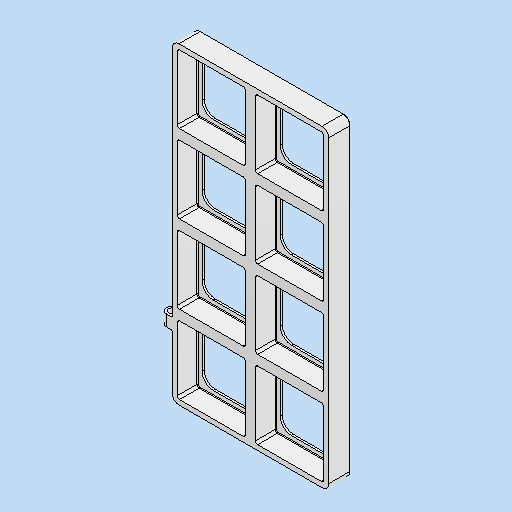
# Autodesk Inventor part: SampleCell
Saved by Autodesk Inventor 2025 (Build 290162000, 162)
## iProperties
Created: 2024-10-28
Part Number: SampleCell
Material: ABS Plastic
Document SubType Name: Modeling
Designer: kuzmin
Density: 1.06 g/cm^3
Appearance: Smooth - White
Author: kuzmin
Autodesk Inventor part; units mm, degrees
ref_plane "YZ Plane" through (0, 0, 0) normal (1, 0, 0) x (0, 1, 0)
ref_plane "XZ Plane" through (0, 0, 0) normal (0, 1, 0) x (-1, 0, 0)
sketch "Sketch1" plane through (0, 0, 0) normal (0, 0, 1) x (-1, 0, 0)
  line L0 (17.5, 17.5) -> (-17.5, 17.5)
  line L1 (-17.5, 17.5) -> (-17.5, -17.5)
  line L2 (-17.5, -17.5) -> (17.5, -17.5)
  line L3 (17.5, -17.5) -> (17.5, 17.5)
  point P0 (0, 0)
  point P1 (17.5, 0)
  point P2 (0, -17.5)
  dimension "d0" = 35
  constraints: 8 end point, 2 midpoint, 2 parallel, 2 perpendicular, 1 horizontal, 1 horizontal alignment, 1 vertical alignment
  measures "d0" distance of L2.end L0.start
extrude "Extrusion1" add sketch "Sketch1" along normal blind 10
sketch "Sketch2" plane through (0, 0, 10) normal (0, 0, 1) x (1, 0, 0)
  line L0 (-15.25, -15.25) -> (15.25, -15.25)
  line L1 (15.25, -15.25) -> (15.25, 15.25)
  line L2 (15.25, 15.25) -> (-15.25, 15.25)
  line L3 (-15.25, 15.25) -> (-15.25, -15.25)
  point P0 (0, 0)
  point P1 (-15.25, 0)
  point P2 (0, 15.25)
  dimension "d3" = 30.5
  constraints: 8 end point, 2 midpoint, 2 parallel, 2 perpendicular, 1 horizontal, 1 horizontal alignment, 1 vertical alignment
  measures "d3" distance of L2.end L0.start
extrude "Extrusion2" cut sketch "Sketch2" against normal through all
sketch "Sketch3" plane through (0, 0, 0) normal (0, 0, -1) x (1, 0, 0)
  line L0 (15.25, 15.25) -> (15.25, -15.25) projected
  line L1 (-15.25, 15.25) -> (15.25, 15.25) projected
  line L2 (-15.25, -15.25) -> (-15.25, 15.25) projected
  line L3 (15.25, -15.25) -> (-15.25, -15.25) projected
  line L4 (13.25, 13.25) -> (-13.25, 13.25)
  line L5 (-13.25, 13.25) -> (-13.25, -13.25)
  line L6 (-13.25, -13.25) -> (13.25, -13.25)
  line L7 (13.25, -13.25) -> (13.25, 13.25)
  point P0 (0, 0)
  point P1 (13.25, 0)
  point P2 (0, -13.25)
  dimension "d6" = 2
  constraints: 8 end point, 2 midpoint, 2 parallel, 2 perpendicular, 1 horizontal, 1 horizontal alignment, 1 vertical alignment
  measures "d6" distance between parallel lines of L0 L7
extrude "Extrusion3" add sketch "Sketch3" against normal blind 0.9
fillet "Fillet1" radius 1 4 edges at (-15.25, -15.25, 5.45) (-15.25, 15.25, 5.45) (15.25, 15.25, 5.45) (15.25, -15.25, 5.45)
fillet "Fillet2" radius 5 4 edges at (-13.25, -13.25, 0.45) (-13.25, 13.25, 0.45) (13.25, 13.25, 0.45) (13.25, -13.25, 0.45)
chamfer "Chamfer1" distance 0.3 angle 45 8 edges at (0, 15.25, 0.9) (14.9571, 14.9571, 0.9) (15.25, 0, 0.9) (14.9571, -14.9571, 0.9) (0, -15.25, 0.9) (-14.9571, -14.9571, 0.9) (-15.25, 0, 0.9) (-14.9571, 14.9571, 0.9)
pattern_linear "Rectangular Pattern1" count 2 spacing 35 along (1, 0, 0) count 4 spacing 35 along (0, 1, 0)
fillet "Fillet4" radius 3 4 edges at (52.5, 122.5, 5) (-17.5, 122.5, 5) (52.5, -17.5, 5) (-17.5, -17.5, 5)
chamfer "Chamfer2" distance 0.5 angle 45 8 edges at (17.5, 122.5, 0) (-16.6213, 121.6213, 0) (-17.5, 52.5, 0) (-16.6213, -16.6213, 0) (17.5, -17.5, 0) (51.6213, -16.6213, 0) (52.5, 52.5, 0) (51.6213, 121.6213, 0)
ref_plane "Work Plane2" through (-14.5, 12.5, 10) normal (0, -1, 0) x (1, 0, 0)
ref_plane "Work Plane1" through (-14.5, 52.5, 10) normal (0, -1, 0) x (1, 0, 0)
sketch "Sketch4" plane through (-14.5, 12.5, 10) normal (0, -1, 0) x (1, 0, 0)
  line L0 (-3, 0) -> (-3, -9.5) projected
  line L1 (-3, -9.5) -> (-8, -3.5412)
  line L2 (-8, -3.5412) -> (-8, 0)
  line L3 (-8, 0) -> (-3, 0)
  circle A0 centre (-5.5, -2.5) radius 1.6
  point P0 (14.5, -10)
  point P1 (-5.5, 0)
  dimension "d35" = 3.2
  dimension "d36" = 5
  dimension "d38" = 40
  dimension "d39" = 2.5
  constraints: 6 end point, 1 centre point, 1 midpoint, 1 parallel, 1 perpendicular, 1 vertical alignment
  measures "d35" diameter of A0
  measures "d36" distance of L2.end L0.start
  measures "d38" angle of L0 L1
  measures "d39" distance from line of L3 A0.centre
extrude "Extrusion5" add sketch "Sketch4" along normal mid plane 5
fillet "Fillet6" radius 2.4 2 edges at (-22.5, 12.5, 10) (-22.5, 12.5, 6.4588)
fillet "Fillet7" radius 0.4 2 edges at (-17.5, 10, 5.25) (-17.5, 15, 5.25)
body "Solid1"
